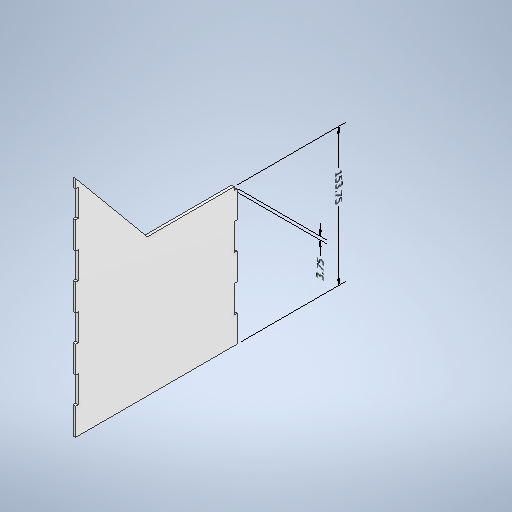
# Autodesk Inventor part: Q side 1
Saved by Autodesk Inventor 2025.3 (Build 293356000, 356)
## iProperties
Created: 2026-04-17
Part Number: Q side 1
Material: ABS Plastic
Document SubType Name: Modeling
Designer: logien
Density: 1.06 g/cm^3
Appearance: Smooth - White
Author: logien
Autodesk Inventor part; units mm, degrees
ref_plane "YZ Plane" through (0, 0, 0) normal (1, 0, 0) x (0, 1, 0)
ref_plane "XZ Plane" through (0, 0, 0) normal (0, 1, 0) x (-1, 0, 0)
ref_plane "XY Plane" through (0, 0, 0) normal (0, 0, 1) x (1, 0, 0)
sketch "Sketch2" plane through (0, 0, 0) normal (1, 0, 0) x (0, 1, 0)
  line L0 (0, -180) -> (0, 0)
  line L1 (0, 0) -> (30, 0)
  line L2 (30, 0) -> (30, -3)
  line L3 (30, -3) -> (60, -3)
  line L4 (60, -3) -> (60, 0)
  line L5 (60, 0) -> (90, 0)
  line L6 (90, 0) -> (90, -3)
  line L7 (90, -3) -> (120, -3)
  line L8 (120, -3) -> (120, 0)
  line L9 (120, 0) -> (150, 0)
  line L10 (150, 0) -> (150, -3)
  line L11 (150, -3) -> (180, -3)
  line L12 (180, -3) -> (180, 0)
  line L13 (180, 0) -> (210, 0)
  line L14 (210, 0) -> (210, -3)
  line L15 (210, -3) -> (240, -3)
  line L16 (240, -3) -> (240, 0)
  line L17 (240, 0) -> (250, 0)
  line L18 (153.75, -180) -> (153.75, -80)
  line L19 (153.75, -80) -> (250, 0)
  line L20 (0, -90) -> (37, -90) construction
  line L21 (0, -180) -> (30, -180)
  line L22 (30, -180) -> (30, -177)
  line L23 (30, -177) -> (60, -177)
  line L24 (60, -177) -> (60, -180)
  line L25 (60, -180) -> (90, -180)
  line L26 (90, -180) -> (90, -177)
  line L27 (90, -177) -> (120, -177)
  line L28 (120, -177) -> (120, -180)
  line L29 (120, -180) -> (150, -180)
  line L30 (150, -180) -> (150, -177)
  line L31 (150, -177) -> (153.75, -177)
  line L32 (153.75, -180) -> (180, -180)
  line L33 (153.75, -180) -> (0, -180)
  point P0 (180, -177)
  point P1 (210, -180)
  dimension "d25" = 180
  dimension "d26" = 250
  dimension "d27" = 30
  dimension "d28" = 3
  dimension "d29" = 30
  dimension "d30" = 3
  dimension "d31" = 30
  dimension "d32" = 3
  dimension "d33" = 30
  dimension "d34" = 3
  dimension "d35" = 30
  dimension "d36" = 3
  dimension "d37" = 30
  dimension "d38" = 3
  dimension "d39" = 30
  dimension "d40" = 3
  dimension "d41" = 30
  dimension "d42" = 3
  dimension "d43" = 10
  dimension "d47" = 203
  dimension "d51" = 100
  constraints: 68 end point, 12 point on line, 12 symmetric about line, 10 parallel, 2 perpendicular, 2 vertical, 1 horizontal, 1 midpoint
  measures "d25" distance of L0.start L0.end
  measures "d26" distance of L0.end L17.end
  measures "d27" distance of L0.end L1.end
  measures "d28" distance of L1.end L2.end
  measures "d29" distance of L2.end L3.end
  measures "d30" distance of L3.end L4.end
  measures "d31" distance of L4.end L5.end
  measures "d32" distance of L5.end L6.end
  measures "d33" distance of L6.end L7.end
  measures "d34" distance of L7.end L8.end
  measures "d35" distance of L8.end L9.end
  measures "d36" distance of L9.end L10.end
  measures "d37" distance of L10.end L11.end
  measures "d38" distance of L11.end L12.end
  measures "d39" distance of L12.end L13.end
  measures "d40" distance of L13.end L14.end
  measures "d41" distance of L14.end L15.end
  measures "d42" distance of L15.end L16.end
  measures "d43" distance of L16.end L17.end
  measures "d47" distance from line of L20.end L16
  measures "d51" distance of L18.start L18.end
extrude "Extrusion2" add sketch "Sketch2" along normal blind 3 contours L0 L1 L2 L3 L4 L5 L6 L7 L8 L9 L10 L11 L12 L13 L14 L15 L16 L17 L19 L18 L31 L30 L29 L28 L27 L26 L25 L24 L23 L22 L21
body "Solid2"
